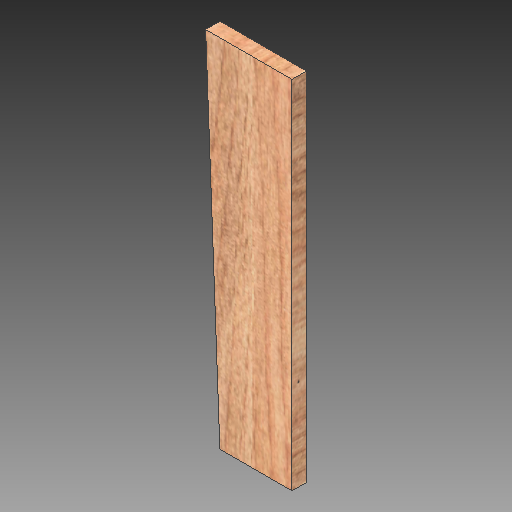
# Autodesk Inventor part: internalSupportTop3
Saved by Autodesk Inventor 2019 (Build 230136000, 136)
## iProperties
Company: FABLAB Torino
Created: 2019-01-11
Part Number: internalSupportTop3
Material: Wood (Birch)
Document SubType Name: Modeling
Designer: Giancarlo
Density: 0.55 g/cm^3
Appearance: Birch - Natural Polished
Description: MultiLayer 10mm
Author: Giancarlo
Title: La Panca - Flower Vase
Subject: Construction MOld
Autodesk Inventor part; units mm, degrees
ref_plane "YZ Plane" through (0, 0, 0) normal (1, 0, 0) x (0, 1, 0)
ref_plane "XZ Plane" through (0, 0, 0) normal (0, 1, 0) x (-1, 0, 0)
ref_plane "Work Plane1" through (0, 0, 0) normal (0, 0, 1) x (1, 0, 0)
sketch "Sketch1" plane through (0, 0, 0) normal (0, 0, 1) x (1, 0, 0)
  line L0 (0, 0) -> (0, 3) construction
  line L1 (-50, 3) -> (0, 3) construction
  line L2 (-50, 0) -> (-50, 3) construction
  line L3 (0, 0) -> (-50, 0) construction
  line L4 (149.2687, 0) -> (0, 0) construction
  line L5 (149.2687, 3) -> (149.2687, 0) construction
  line L6 (0, 3) -> (149.2687, 3) construction
  line L7 (161.2496, 3) -> (161.8322, 3) construction
  spline S0 degree 3 poles (161.8322, 3) (161.8322, 2.5) (161.8322, 2) (161.8322, 1) (161.8322, 0.5) (161.8322, 0) knots -0.3 -0.3 -0.3 -0.3 -0.15 -0.15 0 0 0 0 construction
  line L8 (161.8322, 0) -> (161.2496, 0) construction
  line L9 (161.2496, 0) -> (161.2496, 3) construction
  line L10 (-52.9976, -0.1199) -> (-62.8824, 247) construction
  line L11 (-62.8824, 247) -> (-59.8848, 247.1199) construction
  line L12 (-59.8848, 247.1199) -> (-50, 0)
  line L13 (-50, 0) -> (-52.9976, -0.1199) construction
  line L14 (0, 0) -> (-50, 0)
  line L15 (-59.8848, 247.1199) -> (0, 247.1199)
  line L16 (0, 247.1199) -> (0, 0)
  constraints: 34 end point, 6 horizontal, 4 vertical, 2 perpendicular, 1 collinear, 1 vertical alignment, 18 other
extrude "Extrusion1" add sketch "Sketch1" along normal blind 10
body "Solid1"
